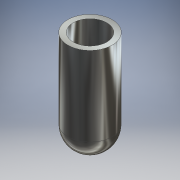
# Autodesk Inventor part: Toggle_Cap
Saved by Autodesk Inventor 2016 (Build 200138000, 138)
## iProperties
Created: 2016-04-13
Part Number: Toggle_Cap
Material: Nickel-Copper Alloy 400
Document SubType Name: Modeling
Designer: agmle
Density: 8.83 g/cm^3
Appearance: Chrome - Polished
Author: agmle
Autodesk Inventor part; units mm, degrees
ref_plane "YZ Plane" through (0, 0, 0) normal (1, 0, 0) x (0, 1, 0)
ref_plane "XZ Plane" through (0, 0, 0) normal (0, 1, 0) x (-1, 0, 0)
ref_plane "XY Plane" through (0, 0, 0) normal (0, 0, 1) x (1, 0, 0)
sketch "Sketch1" plane through (0, 0, 0) normal (0, 1, 0) x (-1, 0, 0)
  line L0 (0, 16) -> (0, 0) construction
  line L1 (2.69, 16) -> (3.55, 16)
  line L2 (3.55, 16) -> (3.55, 3.2798)
  arc A0 (1.3585, 0) -> (3.55, 3.2798) centre (0, 3.2798) ccw
  line L3 (2.69, 16) -> (2.69, 3.2798)
  arc A1 (1.0294, 0.7945) -> (2.69, 3.2798) centre (0, 3.2798) ccw
  line L4 (1.0294, 0.7945) -> (1.3585, 0)
  line L5 (2.69, 16) -> (0, 16) construction
  line L6 (0, 0) -> (3.1469, 0) construction
  dimension "d0" = 16
  dimension "d1" = 22.5
  dimension "d2" = 3.55
  dimension "d3" = 2.69
  constraints: 14 end point, 4 point on circle, 3 perpendicular, 2 centre point, 2 coincident, 2 point on line, 2 tangent, 2 vertical, 1 horizontal, 1 line through centre
  measures "d0" distance of L0.start L0.end
  measures "d1" angle of L0 L4
  measures "d2" distance between parallel lines of L0 L2
  measures "d3" distance between parallel lines of L0 L3
revolve "Revolution1" add sketch "Sketch1" angle 360 about axis through (0, 0, 16) along (0, 0, -1)
body "Solid1"
